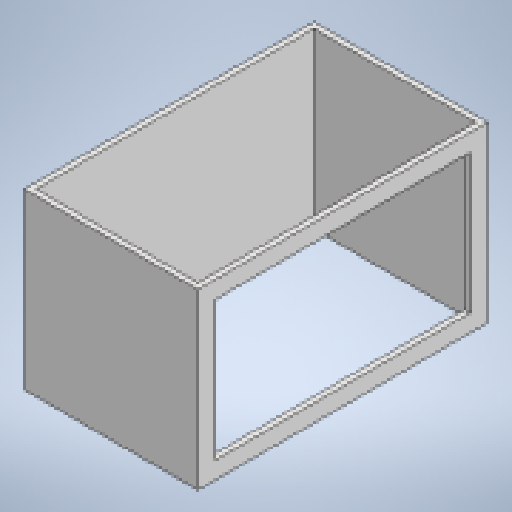
# Autodesk Inventor part: NDM-VOS dummy6
Saved by Autodesk Inventor 2025 (Build 290162010, 162A)
## iProperties
Created: 2024-10-05
Part Number: NDM-VOS dummy6
Material: Generic
Document SubType Name: Modeling
Designer: admin
Density: 1 g/cm^3
Appearance: Default
Author: admin
Autodesk Inventor part; units mm, degrees
ref_plane "YZ Plane" through (0, 0, 0) normal (1, 0, 0) x (0, 1, 0)
ref_plane "XZ Plane" through (0, 0, 0) normal (0, 1, 0) x (-1, 0, 0)
ref_plane "XY Plane" through (0, 0, 0) normal (0, 0, 1) x (1, 0, 0)
sketch "Sketch1" plane through (0, 0, 0) normal (0, 0, 1) x (1, 0, 0)
  line L0 (-150, -250) -> (150, -250)
  line L1 (150, -250) -> (150, 250)
  line L2 (150, 250) -> (-150, 250)
  line L3 (-150, 250) -> (-150, -250)
  line L4 (-150, -250) -> (150, 250) construction
  line L5 (150, -250) -> (-150, 250) construction
  point P0 (0, 0)
  dimension "d0" = 300
  dimension "d1" = 500
  constraints: 12 end point, 2 midpoint, 2 parallel, 1 horizontal, 1 perpendicular
  measures "d0" distance of L2.end L1.end
  measures "d1" distance of L1.end L0.end
extrude "Extrusion1" add sketch "Sketch1" along normal blind 300
shell "Shell1" thickness 10 removed faces 2 at (-50, 83.3333, 300) at (-50, 83.3333, 0)
sketch "Sketch2" plane through (0, 0, 0) normal (1, 0, 0) x (0, 1, 0)
  line L0 (-250, 0) -> (250, 0) construction
  line L1 (250, 0) -> (250, 300) construction
  line L2 (-250, 300) -> (250, 300) construction
  line L3 (-250, 0) -> (-250, 300) construction
  line L4 (-250, 0) -> (-250, 300) construction
  line L5 (-250, 150) -> (250, 150) construction
  circle A0 centre (0, 150) radius 30
  arc A1 (205, 115) -> (17.4379, 125.5885) centre (104.6273, 3.5311) ccw
  arc A2 (160.6867, 200) -> (-12.382, 177.3256) centre (111.438, -95.93) ccw
  arc A3 (205, 115) -> (160.6867, 200) centre (150.8369, 140.814) ccw
  point P0 (0, 0)
  dimension "d5" = 60
  dimension "d6" = 300
  dimension "d7" = 150
  dimension "d8" = 60
  dimension "d9" = 35
  dimension "d10" = 205
  dimension "d11" = 50
  constraints: 8 point on circle, 4 centre point, 3 midpoint, 3 tangent, 2 end point
  measures "d5" diameter of A0
  measures "d6" radius of A2
  measures "d7" radius of A1
  measures "d8" radius of A3
  measures "d9" vertical distance of A1.start A0.centre
  measures "d10" horizontal distance of A0.centre A1.start
  measures "d11" distance from line of L5 A2.start
extrude "Extrusion2" [suppressed]
pattern_linear "Rectangular Pattern1" [suppressed]
pattern_circular "Circular Pattern1" [suppressed]
sketch "Sketch3" plane through (150, -250, 0) normal (1, 0, 0) x (0, 0, -1)
  line L0 (0, 0) -> (0, 500) projected
  line L1 (0, 500) -> (-300, 500) projected
  line L2 (-300, 0) -> (-300, 500) projected
  line L3 (0, 0) -> (-300, 0) projected
  line L4 (-270, 470) -> (-30, 470)
  line L5 (-30, 470) -> (-30, 30)
  line L6 (-30, 30) -> (-270, 30)
  line L7 (-270, 30) -> (-270, 470)
  point P0 (0, 250)
  dimension "d20" = 30
  constraints: 8 end point, 3 other
  measures "d20" distance between parallel lines of L2 L7
extrude "Extrusion3" cut sketch "Sketch3" against normal up to surface (10 mm away) contours L4 L5 L6 L7
body "Solid1"
